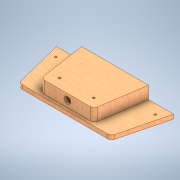
# Autodesk Inventor part: Pont_arriere
Saved by Autodesk Inventor 2021 (Build 250183000, 183)
## iProperties
Created: 2021-05-21
Part Number: Pont_arriere
Material: Bois (Cerisier)
Document SubType Name: Modeling
Designer: dimercur
Density: 0.63 g/cm^3
Appearance: Cerisier - Faible lustre naturel
Author: dimercur
Autodesk Inventor part; units mm, degrees
ref_plane "YZ Plane" through (0, 0, 0) normal (1, 0, 0) x (0, 1, 0)
ref_plane "XZ Plane" through (0, 0, 0) normal (0, 1, 0) x (-1, 0, 0)
ref_plane "XY Plane" through (0, 0, 0) normal (0, 0, 1) x (1, 0, 0)
sketch "Esquisse1" plane through (0, 0, 0) normal (0, 1, 0) x (-1, 0, 0)
  line L0 (55, 30) -> (-55, 30)
  line L1 (-55, 30) -> (-70, -30)
  line L2 (-70, -30) -> (70, -30)
  line L3 (70, -30) -> (55, 30)
  point P0 (0, 0)
  dimension "d0" = 140
  dimension "d1" = 110
  dimension "d2" = 60
  dimension "d3" = 70
  dimension "d4" = 55
  dimension "d5" = 30
  constraints: 8 end point, 1 horizontal, 1 parallel
  measures "d0" distance of L1.end L2.end
  measures "d1" distance of L0.start L0.end
  measures "d2" distance between parallel lines of L2 L0
  measures "d3" horizontal distance of point (0, 0) L2.end
  measures "d4" horizontal distance of point (0, 0) L0.start
  measures "d5" vertical distance of point (0, 0) L2.end
extrude "Extrusion1" add sketch "Esquisse1" along normal blind 5
sketch "Esquisse2" plane through (0, 5, 0) normal (0, 1, 0) x (1, 0, 0)
  line L0 (-31.5, -27) -> (31.5, -27)
  line L1 (31.5, -27) -> (40, 30)
  line L2 (70, 30) -> (-70, 30) projected
  line L3 (-31.5, -27) -> (-40, 30)
  line L4 (40, 30) -> (-40, 30)
  line L5 (-55, -30) -> (55, -30) projected
  point P0 (0, 0)
  dimension "d8" = 80
  dimension "d9" = 63
  dimension "d10" = 31.5
  dimension "d11" = 40
  dimension "d12" = 3
  constraints: 8 end point, 2 horizontal, 2 point on line
  measures "d8" distance of L1.end L3.end
  measures "d9" distance of L0.start L0.end
  measures "d10" horizontal distance of point (0, 0) L0.start
  measures "d11" horizontal distance of L3.end point (0, 0)
  measures "d12" distance from line of L5 L0.start
extrude "Extrusion2" add sketch "Esquisse2" along normal blind 15
sketch "Esquisse3" plane through (-31.5, 5, 27) normal (0, 0, 1) x (1, 0, 0)
  circle A0 centre (31.5, 8) radius 4
  line L0 (0, 0) -> (0, 15) projected
  line L1 (63, 0) -> (63, 15) projected
  line L2 (71.5, 15) -> (-8.5, 15) projected
  point P0 (31.5, -5)
  dimension "d15" = 31.5
  dimension "d16" = 63
  dimension "d17" = 7
  dimension "d18" = 8
  constraints: 1 centre point
  measures "d15" distance from line of L0 A0.centre
  measures "d16" distance between parallel lines of L1 L0
  measures "d17" distance from line of L2 A0.centre
  measures "d18" diameter of A0
extrude "Extrusion3" cut sketch "Esquisse3" against normal blind 20
fillet "Congé1" radius 5 4 edges at (31.5, 12.5, 27) (-31.5, 12.5, 27) (55, 2.5, 30) (-55, 2.5, 30)
sketch "Esquisse5" plane through (0, 20, 0) normal (0, 1, 0) x (1, 0, 0)
  circle A0 centre (-59.5, 18.5) radius 1.25
  circle A1 centre (59.5, 18.5) radius 1.25
  circle A2 centre (20.5, -16) radius 1.25
  circle A3 centre (-20.5, -16) radius 1.25
  line L0 (-40, 30) -> (-70, 30) projected
  line L1 (70, 30) -> (40, 30) projected
  point P0 (0, 0)
  dimension "d22" = 2.5
  dimension "d23" = 2.5
  dimension "d24" = 2.5
  dimension "d25" = 2.5
  dimension "d26" = 119
  dimension "d27" = 41
  dimension "d28" = 59.5
  dimension "d30" = 20.5
  dimension "d31" = 34.5
  dimension "d32" = 11.5
  dimension "d33" = 11.5
  dimension "d34" = 34.5
  constraints: 4 centre point
  measures "d22" diameter of A0
  measures "d23" diameter of A1
  measures "d24" diameter of A2
  measures "d25" diameter of A3
  measures "d26" distance of A1.centre A0.centre
  measures "d27" distance of A2.centre A3.centre
  measures "d28" horizontal distance of A0.centre point (0, 0)
  measures "d30" horizontal distance of A3.centre point (0, 0)
  measures "d31" vertical distance of A3.centre A0.centre
  measures "d32" distance from line of L0 A0.centre
  measures "d33" distance from line of L1 A1.centre
  measures "d34" vertical distance of A1.centre A2.centre
extrude "Extrusion4" cut sketch "Esquisse5" against normal through all
equation "\"d3\" = 0.5 * d0"
equation "\"d4\" = 0.5 * d1"
equation "\"d5\" = 0.5 * d2"
equation "\"d10\" = 0.5 * d9"
equation "\"d11\" = 0.5 * d8"
equation "\"d15\" = 0.5 * d16"
equation "\"d23\" = d22"
equation "\"d24\" = d22"
equation "\"d25\" = d22"
equation "\"d28\" = 0.5 * d26"
equation "\"d30\" = 0.5 * d27"
equation "\"d33\" = d32"
equation "\"d34\" = d31"
